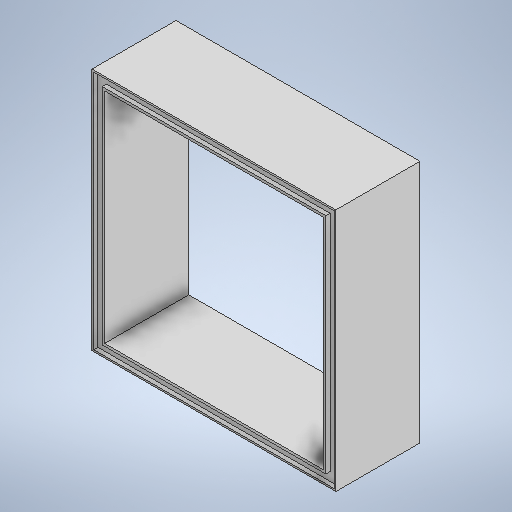
# Autodesk Inventor part: Sweep_0003
Saved by Autodesk Inventor 2025.2 (Build 292293000, 293)
## iProperties
Created: 2025-03-26
Part Number: Sweep_0003
Material: Generic
Document SubType Name: Modeling
Designer: ishad
Density: 1 g/cm^3
Appearance: Default
Author: ishad
Autodesk Inventor part; units mm, degrees
ref_plane "YZ Plane" through (0, 0, 0) normal (1, 0, 0) x (0, 1, 0)
ref_plane "XZ Plane" through (0, 0, 0) normal (0, 1, 0) x (-1, 0, 0)
ref_plane "XY Plane" through (0, 0, 0) normal (0, 0, 1) x (1, 0, 0)
sketch "Sketch1" plane through (0, 0, 0) normal (0, 0, 1) x (1, 0, 0)
  line L0 (12, -12) -> (-12, 12) construction
  line L1 (-12, -12) -> (12, 12) construction
  line L2 (14.5, -14.5) -> (-14.5, -14.5)
  line L3 (-14.5, -14.5) -> (-14.5, 14.5)
  line L4 (-14.5, 14.5) -> (14.5, 14.5)
  line L5 (14.5, 14.5) -> (14.5, -14.5)
  line L6 (14.5, -14.5) -> (-14.5, 14.5) construction
  line L7 (-14.5, -14.5) -> (14.5, 14.5) construction
  line L8 (-13, 13) -> (13, 13)
  line L9 (13, -13) -> (-13, -13)
  line L10 (-13, 13) -> (-13, -13)
  line L11 (13, 13) -> (13, -13)
  point P0 (0, 0)
  dimension "d0" = 29
  dimension "d1" = 29
  dimension "d3" = 26
  constraints: 24 end point, 5 point on line, 4 midpoint, 4 parallel, 2 horizontal, 2 perpendicular
  measures "d0" distance of L3.end L4.end
  measures "d1" distance between parallel lines of L2 L4
  measures "d3" distance of L8.start L9.end
extrude "Extrusion1" add sketch "Sketch1" against normal blind 10
sketch "Sketch5" plane through (0, 0, 0) normal (0, 0, 1) x (1, 0, 0)
  line L0 (-13.5, 0) -> (-13.5, 13.5)
  line L1 (-13.5, 13.5) -> (13.5, 13.5)
  line L2 (13.5, 13.5) -> (13.5, -13.5)
  line L3 (13.5, -13.5) -> (-13.5, -13.5)
  line L4 (-13.5, -13.5) -> (-13.5, 0)
  line L5 (13, 13) -> (-13, 13) projected
  line L6 (13, -13) -> (13, 13) projected
  line L7 (-13, -13) -> (13, -13) projected
  line L8 (-13, 13) -> (-13, -13) projected
  point P0 (0, 0)
  dimension "d11" = 0.5
  dimension "d12" = 0.5
  dimension "d13" = 0.5
  dimension "d14" = 0.5
  constraints: 10 end point, 4 perpendicular, 1 point on line, 1 vertical
  measures "d11" distance between parallel lines of L5 L1
  measures "d12" distance between parallel lines of L2 L6
  measures "d13" distance between parallel lines of L3 L7
  measures "d14" distance between parallel lines of L8 L4
sketch "Sketch6" plane through (0, 0, 0) normal (1, 0, 0) x (0, 1, 0)
  line L0 (13.3, 0.5) -> (14.3, 0.5)
  line L1 (14.3, 0.5) -> (14.3, -0.5)
  line L2 (14.3, -0.5) -> (13.3, -0.5)
  line L3 (13.3, -0.5) -> (13.3, 0.5)
  line L4 (13.3, 0.5) -> (14.3, -0.5) construction
  line L5 (14.3, 0.5) -> (13.3, -0.5) construction
  point P0 (0, 0)
  point P1 (13.8, 0)
  dimension "d15" = 1
  dimension "d16" = 13.8
  constraints: 12 end point, 2 midpoint, 2 parallel, 2 perpendicular, 1 horizontal, 1 horizontal alignment
  measures "d15" distance of L1.end L2.end
  measures "d16" distance of point (13.8, 0) point (0, 0)
sweep "Sweep1" cut profiles "Sketch6" path "Sketch5" path curves L1 L0 L4 L3 L2
equation "\"d12\" = d11"
equation "\"d13\" = d12"
equation "\"d14\" = d11"
body "Solid1"
